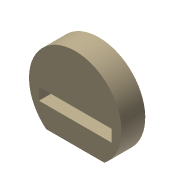
# Autodesk Inventor part: wiper
Saved by Autodesk Inventor 2014 (Build 180170000, 170)
## iProperties
Created: 2015-10-12
Part Number: wiper
Material: Generic
Document SubType Name: Modeling
Designer: Tom
Density: 1 g/cm^3
Appearance: Default
Author: Tom
Autodesk Inventor part; units mm, degrees
ref_plane "YZ Plane" through (0, 0, 0) normal (1, 0, 0) x (0, 1, 0)
ref_plane "XZ Plane" through (0, 0, 0) normal (0, 1, 0) x (-1, 0, 0)
ref_plane "XY Plane" through (0, 0, 0) normal (0, 0, 1) x (1, 0, 0)
sketch "Sketch1" plane through (0, 0, 0) normal (0, 0, 1) x (1, 0, 0)
  arc A0 (1.9352, -2.3876) -> (-1.9352, -2.3876) centre (0, 0) ccw
  line L0 (-1.9352, -2.3876) -> (1.9352, -2.3876)
  line L1 (-2.413, -0.9906) -> (2.413, -0.9906)
  line L2 (2.413, -0.9906) -> (2.413, -0.1944)
  line L3 (2.413, -0.1944) -> (-2.413, -0.1944)
  line L4 (-2.413, -0.1944) -> (-2.413, -0.9906)
  dimension "d0" = 6.1468
  dimension "d1" = 2.3876
  dimension "d2" = 4.826
  dimension "d6" = 1.397
  dimension "d7" = 2.413
  constraints: 10 end point, 2 horizontal, 2 parallel, 2 point on circle, 1 centre point, 1 coincident, 1 perpendicular
  measures "d0" diameter of A0
  measures "d1" vertical distance of point (0, 0) L0.end
  measures "d2" distance of L1.start L1.end
  measures "d6" distance between parallel lines of L1 L0
  measures "d7" horizontal distance of L3.end point (0, 0)
extrude "Extrusion1" add sketch "Sketch1" along normal blind 1.5748
sketch "Sketch3" plane through (0, 0, 0) normal (0, 0, -1) x (-1, 0, 0)
  arc A0 (1.9352, -2.3876) -> (-1.9352, -2.3876) centre (0, 0) ccw projected
  circle A1 centre (0, -1.651) radius 0.3175
  dimension "d13" = 0.635
  dimension "d14" = 1.651
  constraints: 1 centre point
  measures "d13" diameter of A1
  measures "d14" distance of A0.centre A1.centre
extrude "Extrusion3" add sketch "Sketch3" along normal blind 0.381
equation "\"d7\" = 0.5 * d2"
body "Solid1"
